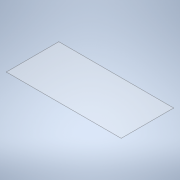
# Autodesk Inventor part: plastic 8 x 17.5
Saved by Autodesk Inventor 2020 (Build 240168000, 168)
## iProperties
Created: 2019-10-11
Part Number: plastic 8 x 17.5
Material: Generic
Document SubType Name: Modeling
Designer: Alex Zaccardelli
Density: 1 g/cm^3
Appearance: Clear - Light
Author: Alex Zaccardelli
Autodesk Inventor part; units mm, degrees
ref_plane "YZ Plane" through (0, 0, 0) normal (1, 0, 0) x (0, 1, 0)
ref_plane "XZ Plane" through (0, 0, 0) normal (0, 1, 0) x (-1, 0, 0)
ref_plane "XY Plane" through (0, 0, 0) normal (0, 0, 1) x (1, 0, 0)
sketch "Sketch1" plane through (0, 0, 0) normal (0, 1, 0) x (-1, 0, 0)
  line L0 (-222.25, 101.6) -> (222.25, 101.6)
  line L1 (222.25, 101.6) -> (222.25, -101.6)
  line L2 (222.25, -101.6) -> (-222.25, -101.6)
  line L3 (-222.25, -101.6) -> (-222.25, 101.6)
  line L4 (-222.25, 101.6) -> (222.25, -101.6) construction
  line L5 (222.25, 101.6) -> (-222.25, -101.6) construction
  point P0 (0, 0)
  dimension "d0" = 444.5
  dimension "d1" = 203.2
  constraints: 12 end point, 2 midpoint, 2 parallel, 1 horizontal, 1 perpendicular
  measures "d0" distance of L1.end L2.end
  measures "d1" distance of L0.end L1.end
extrude "Extrusion1" add sketch "Sketch1" along normal blind 1.016
body "Solid1"
